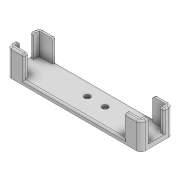
# Autodesk Inventor part: BatteryHolder
Saved by Autodesk Inventor 2022 (Build 260153000, 153)
## iProperties
Created: 2022-11-15
Part Number: BatteryHolder
Material: Generic
Document SubType Name: Modeling
Designer: MVeszpremi
Density: 1 g/cm^3
Appearance: Default
Author: MVeszpremi
Autodesk Inventor part; units mm, degrees
ref_plane "YZ Plane" through (0, 0, 0) normal (1, 0, 0) x (0, 1, 0)
ref_plane "XZ Plane" through (0, 0, 0) normal (0, 1, 0) x (-1, 0, 0)
ref_plane "XY Plane" through (0, 0, 0) normal (0, 0, 1) x (1, 0, 0)
sketch "Sketch1" plane through (0, 0, 0) normal (0, 1, 0) x (-1, 0, 0)
  line L0 (0, 0) -> (142.24, 0)
  line L1 (142.24, 0) -> (142.24, -27.94)
  line L2 (142.24, -27.94) -> (0, -27.94)
  line L3 (0, -27.94) -> (0, 0)
  circle A0 centre (76.1968, -16) radius 1.5
  circle A1 centre (56.1968, -16) radius 1.5
  line L4 (146.24, 4) -> (-4, 4)
  line L5 (-4, 4) -> (-4, -31.94)
  line L6 (-4, -31.94) -> (146.24, -31.94)
  line L7 (146.24, -31.94) -> (146.24, 4)
  line L8 (146.24, -6) -> (-4, -6)
  line L9 (-4, -21.94) -> (146.24, -21.94)
  line L10 (127.24, 4) -> (127.24, -31.94)
  line L11 (15, 4) -> (15, -31.94)
  point P0 (127.24, -27.94)
  point P1 (142.24, -21.94)
  point P2 (127.24, 0)
  point P3 (142.24, -6)
  point P4 (15, -27.94)
  point P5 (0, -21.94)
  point P6 (15, 0)
  point P7 (0, -6)
  dimension "d0" = 142.24
  dimension "d1" = 27.94
  dimension "d2" = 3
  dimension "d3" = 3
  dimension "d4" = 20
  dimension "d7" = 16
  dimension "d8" = 4
  dimension "d9" = 4
  dimension "d10" = 4
  dimension "d11" = 4
  dimension "d12" = 15
  dimension "d13" = 15
  dimension "d14" = 10
  dimension "d15" = 10
  constraints: 24 end point, 8 point on line, 6 perpendicular, 4 parallel, 2 centre point, 2 horizontal, 1 horizontal alignment
  measures "d0" distance of L1.end L2.end
  measures "d1" distance of L0.end L1.end
  measures "d2" diameter of A0
  measures "d3" diameter of A1
  measures "d4" distance of A1.centre A0.centre
  measures "d7" distance from line of L0 A0.centre
  measures "d8" distance between parallel lines of L1 L7
  measures "d9" distance between parallel lines of L4 L0
  measures "d10" distance between parallel lines of L6 L2
  measures "d11" distance between parallel lines of L5 L3
  measures "d12" distance between parallel lines of L3 L11
  measures "d13" distance between parallel lines of L1 L10
  measures "d14" distance between parallel lines of L4 L8
  measures "d15" distance between parallel lines of L6 L9
extrude "Extrusion1" add sketch "Sketch1" along normal blind 5
extrude "Extrusion2" add sketch "Sketch1" along normal blind 30 contours L3 L8 L5 L4 L11 L0 | L10 L4 L7 L8 L1 L0 | L3 L2 L11 L6 L5 L9 | L9 L7 L6 L10 L2 L1
sketch "Sketch2" plane through (0, 5, 0) normal (0, 1, 0) x (1, 0, 0)
  circle A0 centre (-56.1968, 16) radius 1.5 projected
  circle A1 centre (-76.1968, 16) radius 1.5 projected
  line L0 (-146.24, 6) -> (-142.24, 6) projected
  line L1 (-142.24, 6) -> (-142.24, 0) projected
  line L2 (-142.24, 0) -> (-127.24, 0) projected
  line L3 (-127.24, 0) -> (-127.24, -4) projected
  line L4 (-127.24, -4) -> (-15, -4) projected
  line L5 (-15, -4) -> (-15, 0) projected
  line L6 (-15, 0) -> (0, 0) projected
  line L7 (0, 0) -> (0, 6) projected
  line L8 (0, 6) -> (4, 6) projected
  line L9 (4, 6) -> (4, 21.94) projected
  line L10 (4, 21.94) -> (0, 21.94) projected
  line L11 (0, 21.94) -> (0, 27.94) projected
  line L12 (0, 27.94) -> (-15, 27.94) projected
  line L13 (-15, 27.94) -> (-15, 31.94) projected
  line L14 (-15, 31.94) -> (-127.24, 31.94) projected
  line L15 (-127.24, 31.94) -> (-127.24, 27.94) projected
  line L16 (-127.24, 27.94) -> (-142.24, 27.94) projected
  line L17 (-142.24, 27.94) -> (-142.24, 21.94) projected
  line L18 (-142.24, 21.94) -> (-146.24, 21.94) projected
  line L19 (-146.24, 21.94) -> (-146.24, 6) projected
  circle A2 centre (-76.1968, 16) radius 3.25
  circle A3 centre (-56.1968, 16) radius 3.25
  dimension "d20" = 6.5
  dimension "d21" = 6.5
  constraints: 2 centre point, 2 coincident
  measures "d20" diameter of A2
  measures "d21" diameter of A3
extrude "Extrusion3" cut sketch "Sketch2" against normal blind 3.25 contours A0 | A2 | A3
fillet "Fillet1" radius 5 4 edges at (-146.24, 15, -31.94) (-146.24, 15, 4) (4, 15, -31.94) (4, 15, 4)
fillet "Fillet2" radius 2 12 edges at (-144.7755, 30, 2.5355) (-146.24, 30, -3.5) (-134.24, 30, 4) (-144.7755, 30, -30.4755) (-146.24, 30, -24.44) (-134.24, 30, -31.94) (4, 30, -24.44) (-8, 30, -31.94) (2.5355, 30, -30.4755) (-8, 30, 4) (4, 30, -3.5) (2.5355, 30, 2.5355)
fillet "Fillet3" radius 2 26 edges at (-71.12, 5, 4) (-71.12, 5, -31.94) (-127.24, 29.4142, -31.3542) (-127.24, 30, -28.94) (-127.24, 16.5, -31.94) (-127.24, 29.4142, 3.4142) (-127.24, 30, 1) (-127.24, 16.5, 4) (-15, 29.4142, 3.4142) (-15, 30, 1) (-15, 16.5, 4) (-15, 29.4142, -31.3542) (-15, 30, -28.94) (-15, 16.5, -31.94) (3.4142, 29.4142, -6) (1, 30, -6) (4, 16.5, -6) (3.4142, 29.4142, -21.94) (1, 30, -21.94) (4, 16.5, -21.94) (-145.6542, 29.4142, -21.94) (-143.24, 30, -21.94) (-146.24, 16.5, -21.94) (-145.6542, 29.4142, -6) (-143.24, 30, -6) (-146.24, 16.5, -6)
body "Solid1"
